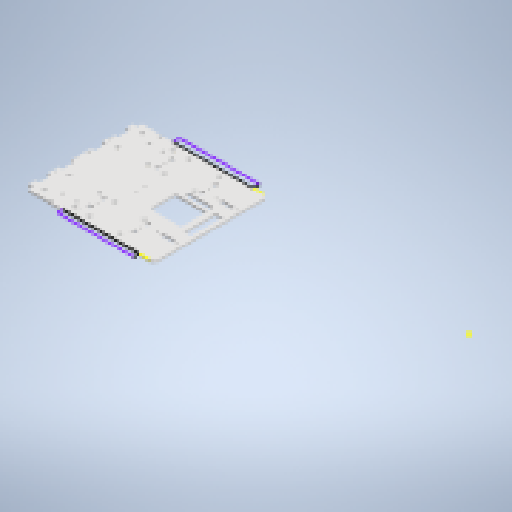
# Autodesk Inventor part: нижняя пластина
Saved by Autodesk Inventor 2024.2 (Build 282272000, 272)
## iProperties
Created: 2025-11-23
Part Number: нижняя пластина
Material: Типовые
Document SubType Name: Modeling
Designer: katya_notebook
Density: 1 g/cm^3
Appearance: По умолчанию
Author: katya_notebook
Autodesk Inventor part; units mm, degrees
(part 1 of 2)
ref_plane "YZ Plane" through (0, 0, 0) normal (1, 0, 0) x (0, 1, 0)
ref_plane "XZ Plane" through (0, 0, 0) normal (0, 1, 0) x (-1, 0, 0)
ref_plane "XY Plane" through (0, 0, 0) normal (0, 0, 1) x (1, 0, 0)
ref_plane "РабПлоскость1" through (-553.2789, -264.3002, 1.4222) normal (0, 1, 0) x (-1, 0, 0)
sketch "Эскиз1" plane through (-553.2789, -264.3002, 1.4222) normal (0, 1, 0) x (-1, 0, 0)
  line L0 (-30, 163.5) -> (30, 163.5) projected
  line L1 (-30, -31.5) -> (30, -31.5) projected
  line L2 (46.4763, 163.5) -> (-176.5237, 163.5)
  line L3 (-176.5237, 163.5) -> (-176.5237, -31.5)
  line L4 (-176.5237, -31.5) -> (46.4763, -31.5)
  line L5 (46.4763, -31.5) -> (46.4763, 163.5)
  point P0 (-553.2789, -1.4222)
  point P1 (-30, -30)
  point P2 (30, -30)
  point P3 (30, 162)
  point P4 (-30, 162)
  dimension "d23" = 8
  dimension "d24" = 8
  dimension "d1" = 223
  dimension "d6" = 0
  dimension "d7" = 0
  constraints: 8 end point, 2 coincident, 2 parallel, 1 horizontal, 1 perpendicular, 1 vertical
  measures "d1" distance of L2.start L2.end
  measures "d6" distance from line of L4 L1.end
  measures "d7" distance from line of L2 L0.end
extrude "Выдавливание1" add sketch "Эскиз1" along normal blind 4
sketch "Эскиз2" plane through (-553.2789, -264.3002, 1.4222) normal (0, -1, 0) x (1, 0, 0)
  circle A0 centre (26, 23.5) radius 2 projected
  circle A1 centre (-26, -19) radius 2 projected
  circle A2 centre (26, -19) radius 2
  circle A3 centre (-26, 23.5) radius 2 projected
  circle A4 centre (-26, -19) radius 2
  point P0 (553.2789, -1.4222)
  dimension "d23" = 8
  dimension "d24" = 8
  constraints: 2 centre point, 1 coincident, 1 concentric
extrude "Выдавливание2" cut sketch "Эскиз2" against normal blind 4
sketch "Эскиз7" plane through (-553.2789, -264.3002, 1.4222) normal (0, -1, 0) x (1, 0, 0)
  line L0 (30, 103.5) -> (30, 157) projected
  line L1 (-46.4763, 163.5) -> (176.5237, 163.5) projected
  line L2 (30.2701, 167.7701) -> (146.6973, 167.7701)
  line L3 (146.803, 163.5) -> (146.803, 157) projected
  line L4 (146.803, 167.7701) -> (146.6973, 167.7701)
  line L5 (146.803, 163.5) -> (30, 163.5)
  line L6 (30, 28.5) -> (30, -25) projected
  line L7 (30, -25) -> (30, -31.5) projected
  line L8 (146.803, -31.5) -> (146.803, -25) projected
  line L9 (146.803, -35.5) -> (30, -35.5)
  line L10 (30, -31.5) -> (146.803, -31.5)
  line L11 (30, 163.5) -> (26, 163.5)
  arc A0 (26, 163.5) -> (30.2701, 167.7701) centre (22.8966, 170.8735) ccw
  line L12 (146.803, 163.5) -> (150.803, 163.5)
  arc A1 (146.803, 167.7701) -> (150.803, 163.5) centre (154.2371, 170.7254) ccw
  line L13 (30, -31.5) -> (26, -31.5)
  line L14 (176.5237, -31.5) -> (-46.4763, -31.5) projected
  arc A2 (30, -35.5) -> (26, -31.5) centre (22.7085, -38.7915) ccw
  line L15 (146.803, -31.5) -> (150.803, -31.5)
  arc A3 (150.803, -31.5) -> (146.803, -35.5) centre (154.0945, -38.7915) ccw
  point P0 (553.2789, -1.4222)
  dimension "d23" = 8
  dimension "d24" = 8
  dimension "d26" = 8
  dimension "d28" = 8
  constraints: 18 end point, 8 point on circle, 5 point on line, 4 centre point, 2 collinear, 1 parallel
  measures "d23" radius of A0
  measures "d24" radius of A1
  measures "d26" radius of A2
  measures "d28" radius of A3
extrude "Выдавливание7" add sketch "Эскиз7" against normal blind 4
sketch "Эскиз10" plane through (-553.2789, -264.3002, 1.4222) normal (0, -1, 0) x (1, 0, 0)
  line L0 (36.9737, 147.85) -> (34.9737, 147.85)
  line L1 (36.9737, 147.85) -> (36.9737, 152.65)
  line L2 (35.9737, 147.85) -> (35.9737, 152.65)
  line L3 (36.9737, 159.35) -> (34.9737, 159.35)
  line L4 (36.9737, 150.25) -> (34.9737, 150.25)
  line L5 (36.9737, 159.35) -> (36.9737, 164.15)
  line L6 (36.9737, 161.75) -> (33.9943, 161.75)
  line L7 (33.9943, 161.75) -> (35.9737, 159.35)
  line L8 (35.9737, 164.15) -> (35.9737, 159.35)
  circle A0 centre (35.9737, 161.75) radius 1
  circle A1 centre (35.9737, 150.25) radius 1
  point P0 (553.2789, -1.4222)
  point P1 (34.9737, 147)
  point P2 (30, 163.5)
  point P3 (34.9737, 161.75)
  point P4 (35.9737, 162.75)
  point P5 (35.9737, 161.75)
  dimension "d23" = 8
  dimension "d24" = 8
  constraints: 18 end point, 4 midpoint, 4 perpendicular, 2 horizontal, 1 horizontal alignment, 6 other
extrude "Выдавливание10" cut sketch "Эскиз10" against normal blind 10 contours A1 L2 L4 | L4 L2 A1 | A1 L4 L2 | L4 A1 L2 | A0 L8 L6 | L6 L8 A0 | A0 L6 L8 | L6 A0 L8
sketch "Эскиз12" plane through (-553.2789, -264.3002, 1.4222) normal (0, -1, 0) x (1, 0, 0)
  circle A0 centre (55.5487, 57.8539) radius 2 projected
  circle A1 centre (55.5487, 73.8539) radius 2 projected
  point P0 (553.2789, -1.4222)
  dimension "d23" = 8
  dimension "d24" = 8
extrude "Выдавливание12" cut sketch "Эскиз12" against normal blind 10
sketch "Эскиз13" plane through (-553.2789, -264.3002, 1.4222) normal (0, -1, 0) x (1, 0, 0)
  point P0 (553.2789, -1.4222)
  dimension "d23" = 8
  dimension "d24" = 8
sketch "Эскиз15" plane through (-553.2789, -264.3002, 1.4222) normal (0, -1, 0) x (1, 0, 0)
  line L0 (169.5237, 93.5765) -> (157.5237, 93.5765)
  line L1 (157.5237, 93.5765) -> (157.5237, 38.5765)
  line L2 (157.5237, 38.5765) -> (169.5237, 38.5765)
  line L3 (169.5237, 38.5765) -> (169.5237, 93.5765)
  line L4 (169.5237, 93.5765) -> (157.5237, 38.5765) construction
  line L5 (157.5237, 93.5765) -> (169.5237, 38.5765) construction
  line L6 (176.5237, 163.5) -> (176.5237, -31.5) projected
  point P0 (553.2789, -1.4222)
  point P1 (163.5237, 66.0765)
  dimension "d23" = 8
  dimension "d24" = 8
  dimension "d57" = 13
  dimension "d58" = 12
  dimension "d59" = 55
  constraints: 12 end point, 2 midpoint, 2 parallel, 1 horizontal, 1 perpendicular
  measures "d57" distance from line of point (163.524, 66.076) L6
  measures "d58" distance of L0.start L0.end
  measures "d59" distance of L0.end L1.end
extrude "Выдавливание14" cut sketch "Эскиз15" against normal blind 10
sketch "Эскиз17" plane through (-553.2789, -260.3002, 1.4222) normal (0, 1, 0) x (1, 0, 0)
  line L0 (-46.4763, -143.5) -> (-46.4763, -123.5) projected
  line L1 (-46.4763, -143.5) -> (-40.4763, -143.5) projected
  line L2 (-40.4763, -123.5) -> (-40.4763, -143.5) projected
  line L3 (-46.4763, -123.5) -> (-40.4763, -123.5) projected
  line L4 (-46.4763, -103.5) -> (-46.4763, -83.5) projected
  line L5 (-46.4763, -103.5) -> (-40.4763, -103.5) projected
  line L6 (-40.4763, -83.5) -> (-40.4763, -103.5) projected
  line L7 (-46.4763, -83.5) -> (-40.4763, -83.5) projected
  line L8 (-46.4763, -48.5) -> (-46.4763, -28.5) projected
  line L9 (-46.4763, -48.5) -> (-40.4763, -48.5) projected
  line L10 (-40.4763, -28.5) -> (-40.4763, -48.5) projected
  line L11 (-46.4763, -28.5) -> (-40.4763, -28.5) projected
  line L12 (-46.4763, -8.5) -> (-46.4763, 11.5) projected
  line L13 (-46.4763, -8.5) -> (-40.4763, -8.5) projected
  line L14 (-40.4763, 11.5) -> (-40.4763, -8.5) projected
  line L15 (-46.4763, 11.5) -> (-40.4763, 11.5) projected
  circle A0 centre (-43.4763, -113.5) radius 1.75 projected
  circle A1 centre (-43.4763, -76.375) radius 1.75 projected
  circle A2 centre (-43.4763, -55.625) radius 1.75 projected
  circle A3 centre (-43.4763, -18.5) radius 1.75 projected
  point P0 (553.2789, 1.4222)
extrude "Выдавливание16" cut sketch "Эскиз17" against normal blind 10
fillet "Сопряжение1" radius 8 4 edges at (-376.7551, -262.3002, -30.0778) (-376.7551, -262.3002, 164.9222) (-599.7551, -262.3002, -30.0778) (-599.7551, -262.3002, 164.9222)
sketch "Эскиз18" plane through (-599.7551, -264.3002, 104.9222) normal (-1, 0, 0) x (0, 0, 1)
  line L0 (-95, 0) -> (-95, 4) projected
  line L1 (-95, 4) -> (-95, 5) projected
  line L2 (-95, 5) -> (-115, 5) projected
  line L3 (-115, 5) -> (-115, 4) projected
  line L4 (-135, 4) -> (-127, 4) projected
  line L5 (-135, 4) -> (-135, -55.705) projected
  line L6 (-115, -55.705) -> (-135, -55.705) projected
  line L7 (-115, -55.705) -> (-115, -60.705) projected
  line L8 (-115, -60.705) -> (-95, -60.705) projected
  line L9 (-95, -60.705) -> (-95, -55.705) projected
  line L10 (-86.75, -55.705) -> (-95, -55.705) projected
  line L11 (-86.75, -55.705) -> (-86.75, -54.205) projected
  line L12 (-86.75, -54.205) -> (-88.25, -54.205) projected
  line L13 (-88.25, -54.205) -> (-88.25, -51.205) projected
  line L14 (-88.25, -51.205) -> (-86.75, -51.205) projected
  line L15 (-86.75, -51.205) -> (-86.75, -43.705) projected
  line L16 (-86.75, -43.705) -> (-83.25, -43.705) projected
  line L17 (-83.25, -43.705) -> (-83.25, -51.205) projected
  line L18 (-83.25, -51.205) -> (-81.75, -51.205) projected
  line L19 (-81.75, -51.205) -> (-81.75, -54.205) projected
  line L20 (-81.75, -54.205) -> (-83.25, -54.205) projected
  line L21 (-83.25, -54.205) -> (-83.25, -55.705) projected
  line L22 (-75, -55.705) -> (-83.25, -55.705) projected
  line L23 (-75, -55.705) -> (-75, -60.705) projected
  line L24 (-75, -60.705) -> (-55, -60.705) projected
  line L25 (-55, -60.705) -> (-55, -55.705) projected
  line L26 (-49.625, -55.705) -> (-55, -55.705) projected
  line L27 (-49.625, -55.705) -> (-49.625, -54.205) projected
  line L28 (-49.625, -54.205) -> (-51.125, -54.205) projected
  line L29 (-51.125, -54.205) -> (-51.125, -51.205) projected
  line L30 (-51.125, -51.205) -> (-49.625, -51.205) projected
  line L31 (-49.625, -51.205) -> (-49.625, -49.705) projected
  line L32 (-49.625, -49.705) -> (-49.625, -49.705) projected
  line L33 (-49.625, -49.705) -> (-49.625, -43.705) projected
  line L34 (-49.625, -43.705) -> (-46.125, -43.705) projected
  line L35 (-46.125, -43.705) -> (-46.125, -51.205) projected
  line L36 (-46.125, -51.205) -> (-44.625, -51.205) projected
  line L37 (-44.625, -51.205) -> (-44.625, -54.205) projected
  line L38 (-44.625, -54.205) -> (-46.125, -54.205) projected
  line L39 (-46.125, -54.205) -> (-46.125, -55.705) projected
  line L40 (-28.875, -55.705) -> (-46.125, -55.705) projected
  line L41 (-28.875, -55.705) -> (-28.875, -54.205) projected
  line L42 (-28.875, -54.205) -> (-30.375, -54.205) projected
  line L43 (-30.375, -54.205) -> (-30.375, -51.205) projected
  line L44 (-30.375, -51.205) -> (-28.875, -51.205) projected
  line L45 (-28.875, -51.205) -> (-28.875, -43.705) projected
  line L46 (-28.875, -43.705) -> (-25.375, -43.705) projected
  line L47 (-25.375, -43.705) -> (-25.375, -51.205) projected
  line L48 (-25.375, -51.205) -> (-23.875, -51.205) projected
  line L49 (-23.875, -51.205) -> (-23.875, -54.205) projected
  line L50 (-23.875, -54.205) -> (-25.375, -54.205) projected
  line L51 (-25.375, -54.205) -> (-25.375, -55.705) projected
  line L52 (-20, -55.705) -> (-25.375, -55.705) projected
  line L53 (-20, -55.705) -> (-20, -60.705) projected
  line L54 (-20, -60.705) -> (0, -60.705) projected
  line L55 (0, -60.705) -> (0, -55.705) projected
  line L56 (8.25, -55.705) -> (0, -55.705) projected
  line L57 (8.25, -55.705) -> (8.25, -54.205) projected
  line L58 (8.25, -54.205) -> (6.75, -54.205) projected
  line L59 (6.75, -54.205) -> (6.75, -51.205) projected
  line L60 (6.75, -51.205) -> (8.25, -51.205) projected
  line L61 (8.25, -51.205) -> (8.25, -43.705) projected
  line L62 (8.25, -43.705) -> (11.75, -43.705) projected
  line L63 (11.75, -43.705) -> (11.75, -51.205) projected
  line L64 (11.75, -51.205) -> (13.25, -51.205) projected
  line L65 (13.25, -51.205) -> (13.25, -54.205) projected
  line L66 (13.25, -54.205) -> (11.75, -54.205) projected
  line L67 (11.75, -54.205) -> (11.75, -55.705) projected
  line L68 (20, -55.705) -> (11.75, -55.705) projected
  line L69 (20, -55.705) -> (20, -60.705) projected
  line L70 (20, -60.705) -> (40, -60.705) projected
  line L71 (40, -60.705) -> (40, -55.705) projected
  line L72 (60, -55.705) -> (40, -55.705) projected
  line L73 (60, 4) -> (60, -55.705) projected
  line L74 (52, 4) -> (60, 4) projected
  line L75 (40, 4) -> (40, 5) projected
  line L76 (40, 5) -> (20, 5) projected
  line L77 (20, 5) -> (20, 4) projected
  line L78 (20, 4) -> (20, 0) projected
  line L79 (20, 0) -> (13.25, 0) projected
  line L80 (13.25, 0) -> (13.25, -0.5) projected
  line L81 (13.25, -0.5) -> (11.75, -0.5) projected
  line L82 (11.75, -0.5) -> (11.75, -8) projected
  line L83 (11.75, -8) -> (8.25, -8) projected
  line L84 (8.25, -8) -> (8.25, -0.5) projected
  line L85 (8.25, -0.5) -> (6.75, -0.5) projected
  line L86 (6.75, -0.5) -> (6.75, 0) projected
  line L87 (6.75, 0) -> (0, 0) projected
  line L88 (0, 0) -> (0, 4) projected
  line L89 (0, 4) -> (0, 5) projected
  line L90 (0, 5) -> (-20, 5) projected
  line L91 (-20, 5) -> (-20, 4) projected
  line L92 (-20, 4) -> (-20, 0) projected
  line L93 (-20, 0) -> (-23.875, 0) projected
  line L94 (-23.875, 0) -> (-23.875, -0.5) projected
  line L95 (-23.875, -0.5) -> (-25.375, -0.5) projected
  line L96 (-25.375, -0.5) -> (-25.375, -8) projected
  line L97 (-25.375, -8) -> (-28.875, -8) projected
  line L98 (-28.875, -8) -> (-28.875, -0.5) projected
  line L99 (-28.875, -0.5) -> (-30.375, -0.5) projected
  line L100 (-30.375, -0.5) -> (-30.375, 0) projected
  line L101 (-30.375, 0) -> (-44.625, 0) projected
  line L102 (-44.625, 0) -> (-44.625, -0.5) projected
  line L103 (-44.625, -0.5) -> (-46.125, -0.5) projected
  line L104 (-46.125, -0.5) -> (-46.125, -8) projected
  line L105 (-46.125, -8) -> (-49.625, -8) projected
  line L106 (-49.625, -8) -> (-49.625, -2) projected
  line L107 (-49.625, -2) -> (-49.625, -2) projected
  line L108 (-49.625, -2) -> (-49.625, -0.5) projected
  line L109 (-49.625, -0.5) -> (-51.125, -0.5) projected
  line L110 (-51.125, -0.5) -> (-51.125, 0) projected
  line L111 (-51.125, 0) -> (-55, 0) projected
  line L112 (-55, 0) -> (-55, 4) projected
  line L113 (-55, 4) -> (-55, 5) projected
  line L114 (-55, 5) -> (-75, 5) projected
  line L115 (-75, 5) -> (-75, 4) projected
  line L116 (-75, 4) -> (-75, 0) projected
  line L117 (-75, 0) -> (-81.75, 0) projected
  line L118 (-81.75, 0) -> (-81.75, -0.5) projected
  line L119 (-81.75, -0.5) -> (-83.25, -0.5) projected
  line L120 (-83.25, -0.5) -> (-83.25, -8) projected
  line L121 (-83.25, -8) -> (-86.75, -8) projected
  line L122 (-86.75, -8) -> (-86.75, -0.5) projected
  line L123 (-86.75, -0.5) -> (-88.25, -0.5) projected
  line L124 (-88.25, -0.5) -> (-88.25, 0) projected
  line L125 (-88.25, 0) -> (-95, 0) projected
  line L126 (52, 0) -> (-127, 0) projected
  line L127 (52, 0) -> (52, 4)
  line L128 (52, 4) -> (60, 4)
  line L129 (60, 0) -> (60, 4)
  line L130 (60, 0) -> (52, 0)
  line L131 (-127, 0) -> (-127, 4)
  line L132 (-135, 0) -> (-135, 4)
  line L133 (-127, 4) -> (-135, 4)
  line L134 (-135, 0) -> (-127, 0)
  line L135 (-127, 0) -> (-127, 4) projected
  line L136 (52, 4) -> (52, 0) projected
  line L137 (52, 0) -> (40, 0) projected
  line L138 (40, 0) -> (40, 4) projected
  line L139 (-115, 4) -> (-115, 0) projected
  line L140 (-115, 0) -> (-127, 0) projected
  line L141 (-86.2339, -29.706) -> (-86.2339, -22.2488) projected
  spline S0 degree 2 poles (-86.2339, -22.2488) (-86.2339, -21.6567) (-85.6418, -21.6567) knots 0 0 0 1 1 1 projected
  spline S1 degree 2 poles (-85.6418, -21.6567) (-85.0497, -21.6567) (-85.0497, -22.2488) knots 0 0 0 1 1 1 projected
  line L142 (-85.0497, -22.2488) -> (-85.0497, -29.1139) projected
  line L143 (-85.0497, -29.1139) -> (-83.6248, -29.1139) projected
  line L144 (-83.6248, -29.1139) -> (-82.052, -22.0545) projected
  spline S2 degree 2 poles (-82.052, -22.0545) (-81.9595, -21.6567) (-81.4968, -21.6567) knots 0 0 0 1 1 1 projected
  spline S3 degree 2 poles (-81.4968, -21.6567) (-80.9047, -21.6567) (-80.9047, -22.2303) knots 0 0 0 1 1 1 projected
  spline S4 degree 2 poles (-80.9047, -22.2303) (-80.9047, -22.3043) (-80.914, -22.3599) knots 0 0 0 1 1 1 projected
  line L145 (-80.914, -22.3599) -> (-82.5886, -29.9003) projected
  spline S5 degree 2 poles (-82.5886, -29.9003) (-82.6811, -30.2889) (-83.153, -30.2889) knots 0 0 0 1 1 1 projected
  line L146 (-83.153, -30.2889) -> (-85.6418, -30.2889) projected
  spline S6 degree 2 poles (-85.6418, -30.2889) (-86.2339, -30.2889) (-86.2339, -29.706) knots 0 0 0 1 1 1 projected
  line L147 (-79.4429, -28.4663) -> (-79.4429, -23.4886) projected
  spline S7 degree 2 poles (-79.4429, -23.4886) (-79.4429, -22.7299) (-78.3696, -21.6567) (-77.611, -21.6567) knots 0 0 0 1 2 2 2 projected
  line L148 (-77.611, -21.6567) -> (-75.9548, -21.6567) projected
  spline S8 degree 2 poles (-75.9548, -21.6567) (-75.1869, -21.6567) (-74.1229, -22.7299) (-74.1229, -23.4886) knots 0 0 0 1 2 2 2 projected
  line L149 (-74.1229, -23.4886) -> (-74.1229, -28.4663) projected
  spline S9 degree 2 poles (-74.1229, -28.4663) (-74.1229, -29.2157) (-75.1962, -30.2889) (-75.9548, -30.2889) knots 0 0 0 1 2 2 2 projected
  line L150 (-75.9548, -30.2889) -> (-77.611, -30.2889) projected
  spline S10 degree 2 poles (-77.611, -30.2889) (-78.3604, -30.2889) (-79.4429, -29.2064) (-79.4429, -28.4663) knots 0 0 0 1 2 2 2 projected
  spline S11 degree 2 poles (-44.951, -30.2704) (-45.2008, -30.2704) (-45.5616, -29.9096) (-45.5616, -29.6783) knots 0 0 0 1 2 2 2 projected
  spline S12 degree 2 poles (-45.5616, -29.6783) (-45.5616, -29.4655) (-45.4043, -29.2897) knots 0 0 0 1 1 1 projected
  spline S13 degree 2 poles (-45.4043, -29.2897) (-44.109, -27.8649) (-42.8785, -26.5603) knots 0 0 0 1 1 1 projected
  line L151 (-42.8785, -26.5603) -> (-45.4506, -22.5542) projected
  spline S14 degree 2 poles (-45.4506, -22.5542) (-45.5431, -22.4061) (-45.5431, -22.2488) knots 0 0 0 1 1 1 projected
  spline S15 degree 2 poles (-45.5431, -22.2488) (-45.5431, -21.999) (-45.173, -21.6567) (-44.9417, -21.6567) knots 0 0 0 1 2 2 2 projected
  spline S16 degree 2 poles (-44.9417, -21.6567) (-44.6364, -21.6567) (-44.4328, -22.0638) knots 0 0 0 1 1 1 projected
  line L152 (-44.4328, -22.0638) -> (-42.1013, -25.7646) projected
  spline S17 degree 2 poles (-42.1013, -25.7646) (-42.0273, -25.5611) (-41.3982, -24.8672) knots 0 0 0 1 1 1 projected
  line L153 (-41.3982, -24.8672) -> (-41.3982, -22.2488) projected
  spline S18 degree 2 poles (-41.3982, -22.2488) (-41.3982, -21.6567) (-40.806, -21.6567) knots 0 0 0 1 1 1 projected
  spline S19 degree 2 poles (-40.806, -21.6567) (-40.2139, -21.6567) (-40.2139, -22.2488) knots 0 0 0 1 1 1 projected
  line L154 (-40.2139, -22.2488) -> (-40.2139, -29.706) projected
  spline S20 degree 2 poles (-40.2139, -29.706) (-40.2139, -30.2889) (-40.806, -30.2889) knots 0 0 0 1 1 1 projected
  spline S21 degree 2 poles (-40.806, -30.2889) (-41.3982, -30.2889) (-41.3982, -29.706) knots 0 0 0 1 1 1 projected
  line L155 (-41.3982, -29.706) -> (-41.3982, -26.3568) projected
  line L156 (-41.3982, -26.3568) -> (-44.4791, -29.9929) projected
  spline S22 degree 2 poles (-44.4791, -29.9929) (-44.7104, -30.2704) (-44.951, -30.2704) knots 0 0 0 1 1 1 projected
  line L157 (-33.6634, -29.7153) -> (-33.6634, -22.2488) projected
  spline S23 degree 2 poles (-33.6634, -22.2488) (-33.6634, -21.6567) (-33.0712, -21.6567) knots 0 0 0 1 1 1 projected
  line L158 (-33.0712, -21.6567) -> (-30.1753, -21.6567) projected
  spline S24 degree 2 poles (-30.1753, -21.6567) (-29.4074, -21.6567) (-28.3434, -22.7299) (-28.3434, -23.4979) knots 0 0 0 1 2 2 2 projected
  line L159 (-28.3434, -23.4979) -> (-28.3434, -29.7153) projected
  spline S25 degree 2 poles (-28.3434, -29.7153) (-28.3434, -30.2982) (-28.9355, -30.2982) knots 0 0 0 1 1 1 projected
  spline S26 degree 2 poles (-28.9355, -30.2982) (-29.5277, -30.2982) (-29.5277, -29.7153) knots 0 0 0 1 1 1 projected
  line L160 (-29.5277, -29.7153) -> (-29.5277, -23.4979) projected
  spline S27 degree 2 poles (-29.5277, -23.4979) (-29.5277, -23.2203) (-29.9163, -22.8317) (-30.1753, -22.8317) knots 0 0 0 1 2 2 2 projected
  line L161 (-30.1753, -22.8317) -> (-32.4791, -22.8317) projected
  line L162 (-32.4791, -22.8317) -> (-32.4791, -29.7153) projected
  spline S28 degree 2 poles (-32.4791, -29.7153) (-32.4791, -30.2982) (-33.0712, -30.2982) knots 0 0 0 1 1 1 projected
  spline S29 degree 2 poles (-33.0712, -30.2982) (-33.6634, -30.2982) (-33.6634, -29.7153) knots 0 0 0 1 1 1 projected
  line L163 (-26.8723, -29.706) -> (-26.8723, -22.2488) projected
  spline S30 degree 2 poles (-26.8723, -22.2488) (-26.8723, -21.6567) (-26.2802, -21.6567) knots 0 0 0 1 1 1 projected
  spline S31 degree 2 poles (-26.2802, -21.6567) (-25.6881, -21.6567) (-25.6881, -22.2488) knots 0 0 0 1 1 1 projected
  line L164 (-25.6881, -22.2488) -> (-25.6881, -29.706) projected
  spline S32 degree 2 poles (-25.6881, -29.706) (-25.6881, -30.2889) (-26.2802, -30.2889) knots 0 0 0 1 1 1 projected
  spline S33 degree 2 poles (-26.2802, -30.2889) (-26.8723, -30.2889) (-26.8723, -29.706) knots 0 0 0 1 1 1 projected
  line L165 (-19.2671, -28.4663) -> (-19.2671, -23.4886) projected
  spline S34 degree 2 poles (-19.2671, -23.4886) (-19.2671, -22.7392) (-18.1938, -21.6567) (-17.4167, -21.6567) knots 0 0 0 1 2 2 2 projected
  line L166 (-17.4167, -21.6567) -> (-15.779, -21.6567) projected
  spline S35 degree 2 poles (-15.779, -21.6567) (-15.0019, -21.6567) (-13.9286, -22.7299) (-13.9286, -23.4886) knots 0 0 0 1 2 2 2 projected
  line L167 (-13.9286, -23.4886) -> (-13.9286, -31.7878) projected
  spline S36 degree 2 poles (-13.9286, -31.7878) (-13.9286, -32.639) (-14.5022, -33.1386) knots 0 0 0 1 1 1 projected
  spline S37 degree 2 poles (-14.5022, -33.1386) (-15.0111, -33.6012) (-15.7605, -33.6012) knots 0 0 0 1 1 1 projected
  spline S38 degree 2 poles (-15.7605, -33.6012) (-16.5007, -33.6012) (-17.0188, -33.1386) knots 0 0 0 1 1 1 projected
  spline S39 degree 2 poles (-17.0188, -33.1386) (-17.5924, -32.6297) (-17.5924, -31.7785) knots 0 0 0 1 1 1 projected
  spline S40 degree 2 poles (-17.5924, -31.7785) (-17.5924, -31.1309) (-17.1668, -30.622) knots 0 0 0 1 1 1 projected
  spline S41 degree 2 poles (-17.1668, -30.622) (-16.8153, -30.3352) (-16.4637, -30.2889) knots 0 0 0 1 1 1 projected
  line L168 (-16.4637, -30.2889) -> (-17.4167, -30.2889) projected
  spline S42 degree 2 poles (-17.4167, -30.2889) (-18.1938, -30.2889) (-19.2671, -29.2157) (-19.2671, -28.4663) knots 0 0 0 1 2 2 2 projected
  line L169 (-12.476, -28.4663) -> (-12.476, -23.4886) projected
  spline S43 degree 2 poles (-12.476, -23.4886) (-12.476, -22.7299) (-11.4028, -21.6567) (-10.6441, -21.6567) knots 0 0 0 1 2 2 2 projected
  line L170 (-10.6441, -21.6567) -> (-8.988, -21.6567) projected
  spline S44 degree 2 poles (-8.988, -21.6567) (-8.22, -21.6567) (-7.1561, -22.7299) (-7.1561, -23.4886) knots 0 0 0 1 2 2 2 projected
  line L171 (-7.1561, -23.4886) -> (-7.1561, -28.4663) projected
  spline S45 degree 2 poles (-7.1561, -28.4663) (-7.1561, -29.2157) (-8.2293, -30.2889) (-8.988, -30.2889) knots 0 0 0 1 2 2 2 projected
  line L172 (-8.988, -30.2889) -> (-10.6441, -30.2889) projected
  spline S46 degree 2 poles (-10.6441, -30.2889) (-11.3935, -30.2889) (-12.476, -29.2064) (-12.476, -28.4663) knots 0 0 0 1 2 2 2 projected
  line L173 (1.0783, -28.4663) -> (1.0783, -23.4886) projected
  spline S47 degree 2 poles (1.0783, -23.4886) (1.0783, -22.7392) (2.1516, -21.6567) (2.9288, -21.6567) knots 0 0 0 1 2 2 2 projected
  line L174 (2.9288, -21.6567) -> (4.5664, -21.6567) projected
  spline S48 degree 2 poles (4.5664, -21.6567) (5.3436, -21.6567) (6.4168, -22.7299) (6.4168, -23.4886) knots 0 0 0 1 2 2 2 projected
  line L175 (6.4168, -23.4886) -> (6.4168, -31.7878) projected
  spline S49 degree 2 poles (6.4168, -31.7878) (6.4168, -32.639) (5.8432, -33.1386) knots 0 0 0 1 1 1 projected
  spline S50 degree 2 poles (5.8432, -33.1386) (5.3343, -33.6012) (4.5849, -33.6012) knots 0 0 0 1 1 1 projected
  spline S51 degree 2 poles (4.5849, -33.6012) (3.8447, -33.6012) (3.3266, -33.1386) knots 0 0 0 1 1 1 projected
  spline S52 degree 2 poles (3.3266, -33.1386) (2.753, -32.6297) (2.753, -31.7785) knots 0 0 0 1 1 1 projected
  spline S53 degree 2 poles (2.753, -31.7785) (2.753, -31.1309) (3.1786, -30.622) knots 0 0 0 1 1 1 projected
  spline S54 degree 2 poles (3.1786, -30.622) (3.5301, -30.3352) (3.8817, -30.2889) knots 0 0 0 1 1 1 projected
  line L176 (3.8817, -30.2889) -> (2.9288, -30.2889) projected
  spline S55 degree 2 poles (2.9288, -30.2889) (2.1516, -30.2889) (1.0783, -29.2157) (1.0783, -28.4663) knots 0 0 0 1 2 2 2 projected
  line L177 (14.6419, -29.706) -> (14.6419, -22.2488) projected
  spline S56 degree 2 poles (14.6419, -22.2488) (14.6419, -21.6567) (15.2341, -21.6567) knots 0 0 0 1 1 1 projected
  spline S57 degree 2 poles (15.2341, -21.6567) (15.8262, -21.6567) (15.8262, -22.2488) knots 0 0 0 1 1 1 projected
  line L178 (15.8262, -22.2488) -> (15.8262, -29.1139) projected
  line L179 (15.8262, -29.1139) -> (17.251, -29.1139) projected
  line L180 (17.251, -29.1139) -> (18.8239, -22.0545) projected
  spline S58 degree 2 poles (18.8239, -22.0545) (18.9164, -21.6567) (19.379, -21.6567) knots 0 0 0 1 1 1 projected
  spline S59 degree 2 poles (19.379, -21.6567) (19.9712, -21.6567) (19.9712, -22.2303) knots 0 0 0 1 1 1 projected
  spline S60 degree 2 poles (19.9712, -22.2303) (19.9712, -22.3043) (19.9619, -22.3599) knots 0 0 0 1 1 1 projected
  line L181 (19.9619, -22.3599) -> (18.2873, -29.9003) projected
  spline S61 degree 2 poles (18.2873, -29.9003) (18.1948, -30.2889) (17.7229, -30.2889) knots 0 0 0 1 1 1 projected
  line L182 (17.7229, -30.2889) -> (15.2341, -30.2889) projected
  spline S62 degree 2 poles (15.2341, -30.2889) (14.6419, -30.2889) (14.6419, -29.706) knots 0 0 0 1 1 1 projected
  line L183 (21.433, -30.9551) -> (21.433, -24.3213) projected
  spline S63 degree 2 poles (21.433, -24.3213) (21.433, -23.2111) (22.9966, -21.6567) (24.1069, -21.6567) knots 0 0 0 1 2 2 2 projected
  line L184 (24.1069, -21.6567) -> (24.9303, -21.6567) projected
  spline S64 degree 2 poles (24.9303, -21.6567) (26.0406, -21.6567) (27.5949, -23.2111) (27.5949, -24.3213) knots 0 0 0 1 2 2 2 projected
  line L185 (27.5949, -24.3213) -> (27.5949, -30.9551) projected
  spline S65 degree 2 poles (27.5949, -30.9551) (27.5949, -32.0561) (26.0406, -33.6104) (24.9303, -33.6104) knots 0 0 0 1 2 2 2 projected
  line L186 (24.9303, -33.6104) -> (24.1069, -33.6104) projected
  spline S66 degree 2 poles (24.1069, -33.6104) (22.9966, -33.6104) (21.433, -32.0561) (21.433, -30.9551) knots 0 0 0 1 2 2 2 projected
  line L187 (7.8694, -29.706) -> (7.8694, -22.2488) projected
  spline S67 degree 2 poles (7.8694, -22.2488) (7.8694, -21.6567) (8.4615, -21.6567) knots 0 0 0 1 1 1 projected
  line L188 (8.4615, -21.6567) -> (11.3574, -21.6567) projected
  spline S68 degree 2 poles (11.3574, -21.6567) (12.1254, -21.6567) (13.1894, -22.7299) (13.1894, -23.4886) knots 0 0 0 1 2 2 2 projected
  line L189 (13.1894, -23.4886) -> (13.1894, -29.706) projected
  spline S69 degree 2 poles (13.1894, -29.706) (13.1894, -30.2889) (12.5972, -30.2889) knots 0 0 0 1 1 1 projected
  spline S70 degree 2 poles (12.5972, -30.2889) (12.0051, -30.2889) (12.0051, -29.706) knots 0 0 0 1 1 1 projected
  line L190 (12.0051, -29.706) -> (12.0051, -23.4979) projected
  spline S71 degree 2 poles (12.0051, -23.4979) (12.0051, -23.2203) (11.6165, -22.8317) (11.3574, -22.8317) knots 0 0 0 1 2 2 2 projected
  line L191 (11.3574, -22.8317) -> (9.0537, -22.8317) projected
  line L192 (9.0537, -22.8317) -> (9.0537, -29.706) projected
  spline S72 degree 2 poles (9.0537, -29.706) (9.0537, -30.2889) (8.4615, -30.2889) knots 0 0 0 1 1 1 projected
  spline S73 degree 2 poles (8.4615, -30.2889) (7.8694, -30.2889) (7.8694, -29.706) knots 0 0 0 1 1 1 projected
  spline S74 degree 2 poles (-5.1113, -30.2704) (-5.3611, -30.2704) (-5.722, -29.9096) (-5.722, -29.6783) knots 0 0 0 1 2 2 2 projected
  spline S75 degree 2 poles (-5.722, -29.6783) (-5.722, -29.4655) (-5.5647, -29.2897) knots 0 0 0 1 1 1 projected
  spline S76 degree 2 poles (-5.5647, -29.2897) (-4.2694, -27.8649) (-3.0389, -26.5603) knots 0 0 0 1 1 1 projected
  line L193 (-3.0389, -26.5603) -> (-5.6109, -22.5542) projected
  spline S77 degree 2 poles (-5.6109, -22.5542) (-5.7035, -22.4061) (-5.7035, -22.2488) knots 0 0 0 1 1 1 projected
  spline S78 degree 2 poles (-5.7035, -22.2488) (-5.7035, -21.999) (-5.3334, -21.6567) (-5.1021, -21.6567) knots 0 0 0 1 2 2 2 projected
  spline S79 degree 2 poles (-5.1021, -21.6567) (-4.7968, -21.6567) (-4.5932, -22.0638) knots 0 0 0 1 1 1 projected
  line L194 (-4.5932, -22.0638) -> (-2.2617, -25.7646) projected
  spline S80 degree 2 poles (-2.2617, -25.7646) (-2.1877, -25.5611) (-1.5585, -24.8672) knots 0 0 0 1 1 1 projected
  line L195 (-1.5585, -24.8672) -> (-1.5585, -22.2488) projected
  spline S81 degree 2 poles (-1.5585, -22.2488) (-1.5585, -21.6567) (-0.9664, -21.6567) knots 0 0 0 1 1 1 projected
  spline S82 degree 2 poles (-0.9664, -21.6567) (-0.3742, -21.6567) (-0.3742, -22.2488) knots 0 0 0 1 1 1 projected
  line L196 (-0.3742, -22.2488) -> (-0.3742, -29.706) projected
  spline S83 degree 2 poles (-0.3742, -29.706) (-0.3742, -30.2889) (-0.9664, -30.2889) knots 0 0 0 1 1 1 projected
  spline S84 degree 2 poles (-0.9664, -30.2889) (-1.5585, -30.2889) (-1.5585, -29.706) knots 0 0 0 1 1 1 projected
  line L197 (-1.5585, -29.706) -> (-1.5585, -26.3568) projected
  line L198 (-1.5585, -26.3568) -> (-4.6395, -29.9929) projected
  spline S85 degree 2 poles (-4.6395, -29.9929) (-4.8708, -30.2704) (-5.1113, -30.2704) knots 0 0 0 1 1 1 projected
  line L199 (-25.2162, -24.7377) -> (-25.2162, -23.4886) projected
  spline S86 degree 2 poles (-25.2162, -23.4886) (-25.2162, -22.7299) (-24.1429, -21.6567) (-23.375, -21.6567) knots 0 0 0 1 2 2 2 projected
  line L200 (-23.375, -21.6567) -> (-21.3025, -21.6567) projected
  spline S87 degree 2 poles (-21.3025, -21.6567) (-20.7104, -21.6567) (-20.7104, -22.2488) knots 0 0 0 1 1 1 projected
  line L201 (-20.7104, -22.2488) -> (-20.7104, -29.706) projected
  spline S88 degree 2 poles (-20.7104, -29.706) (-20.7104, -30.2889) (-21.3025, -30.2889) knots 0 0 0 1 1 1 projected
  spline S89 degree 2 poles (-21.3025, -30.2889) (-21.8947, -30.2889) (-21.8947, -29.706) knots 0 0 0 1 1 1 projected
  line L202 (-21.8947, -29.706) -> (-21.8947, -26.5603) projected
  line L203 (-21.8947, -26.5603) -> (-23.3843, -26.5603) projected
  spline S90 degree 2 poles (-23.3843, -26.5603) (-24.1429, -26.5603) (-25.2162, -25.4778) (-25.2162, -24.7377) knots 0 0 0 1 2 2 2 projected
  spline S91 degree 2 poles (-32.4143, -33.0276) (-32.4143, -32.4354) (-31.8222, -32.4354) knots 0 0 0 1 1 1 projected
  line L204 (-31.8222, -32.4354) -> (-30.1846, -32.4354) projected
  spline S92 degree 2 poles (-30.1846, -32.4354) (-29.5924, -32.4354) (-29.5924, -33.0276) knots 0 0 0 1 1 1 projected
  spline S93 degree 2 poles (-29.5924, -33.0276) (-29.5924, -33.6104) (-30.1846, -33.6104) knots 0 0 0 1 1 1 projected
  line L205 (-30.1846, -33.6104) -> (-31.8222, -33.6104) projected
  spline S94 degree 2 poles (-31.8222, -33.6104) (-32.4143, -33.6104) (-32.4143, -33.0276) knots 0 0 0 1 1 1 projected
  spline S95 degree 2 poles (-52.6765, -22.7762) (-53.0836, -22.6189) (-53.0836, -22.2396) knots 0 0 0 1 1 1 projected
  spline S96 degree 2 poles (-53.0836, -22.2396) (-53.0836, -21.6289) (-52.5007, -21.6289) knots 0 0 0 1 1 1 projected
  spline S97 degree 2 poles (-52.5007, -21.6289) (-52.0658, -21.6289) (-51.631, -22.2118) knots 0 0 0 1 1 1 projected
  spline S98 degree 2 poles (-51.631, -22.2118) (-51.2239, -21.6567) (-50.3912, -21.6567) knots 0 0 0 1 1 1 projected
  line L206 (-50.3912, -21.6567) -> (-48.7351, -21.6567) projected
  spline S99 degree 2 poles (-48.7351, -21.6567) (-47.9672, -21.6567) (-46.9032, -22.7299) (-46.9032, -23.4886) knots 0 0 0 1 2 2 2 projected
  line L207 (-46.9032, -23.4886) -> (-46.9032, -28.4663) projected
  spline S100 degree 2 poles (-46.9032, -28.4663) (-46.9032, -29.2157) (-47.9764, -30.2889) (-48.7351, -30.2889) knots 0 0 0 1 2 2 2 projected
  line L208 (-48.7351, -30.2889) -> (-51.631, -30.2889) projected
  spline S101 degree 2 poles (-51.631, -30.2889) (-52.2231, -30.2889) (-52.2231, -29.706) knots 0 0 0 1 1 1 projected
  line L209 (-52.2231, -29.706) -> (-52.2231, -23.4701) projected
  spline S102 degree 2 poles (-52.2231, -23.4701) (-52.2231, -22.9612) (-52.6765, -22.7762) knots 0 0 0 1 1 1 projected
  line L210 (-59.0975, -28.4663) -> (-59.0975, -23.4886) projected
  spline S103 degree 2 poles (-59.0975, -23.4886) (-59.0975, -22.7392) (-58.0242, -21.6567) (-57.2563, -21.6567) knots 0 0 0 1 2 2 2 projected
  line L211 (-57.2563, -21.6567) -> (-55.6187, -21.6567) projected
  spline S104 degree 2 poles (-55.6187, -21.6567) (-54.8415, -21.6567) (-53.7775, -22.7299) (-53.7775, -23.4886) knots 0 0 0 1 2 2 2 projected
  line L212 (-53.7775, -23.4886) -> (-53.7775, -28.4663) projected
  spline S105 degree 2 poles (-53.7775, -28.4663) (-53.7775, -29.2157) (-54.8415, -30.2889) (-55.6187, -30.2889) knots 0 0 0 1 2 2 2 projected
  line L213 (-55.6187, -30.2889) -> (-56.5716, -30.2889) projected
  line L214 (-56.5716, -30.2889) -> (-54.0828, -32.5557) projected
  spline S106 degree 2 poles (-54.0828, -32.5557) (-53.722, -32.824) (-53.722, -33.0923) knots 0 0 0 1 1 1 projected
  spline S107 degree 2 poles (-53.722, -33.0923) (-53.722, -33.6104) (-54.3696, -33.6104) knots 0 0 0 1 1 1 projected
  line L215 (-54.3696, -33.6104) -> (-58.5053, -33.6104) projected
  spline S108 degree 2 poles (-58.5053, -33.6104) (-59.0975, -33.6104) (-59.0975, -33.0276) knots 0 0 0 1 1 1 projected
  spline S109 degree 2 poles (-59.0975, -33.0276) (-59.0975, -32.4354) (-58.5053, -32.4354) knots 0 0 0 1 1 1 projected
  line L216 (-58.5053, -32.4354) -> (-55.5632, -32.4354) projected
  line L217 (-55.5632, -32.4354) -> (-58.6349, -29.632) projected
  spline S110 degree 2 poles (-58.6349, -29.632) (-59.0975, -29.2157) (-59.0975, -28.4663) knots 0 0 0 1 1 1 projected
  line L218 (-64.0566, -21.6474) -> (-61.7436, -21.6474) projected
  line L219 (-61.7436, -21.6474) -> (-61.7436, -18.9273) projected
  spline S111 degree 2 poles (-61.7436, -18.9273) (-61.7436, -18.3352) (-61.1514, -18.3352) knots 0 0 0 1 1 1 projected
  spline S112 degree 2 poles (-61.1514, -18.3352) (-60.5593, -18.3352) (-60.5593, -18.9273) knots 0 0 0 1 1 1 projected
  line L220 (-60.5593, -18.9273) -> (-60.5593, -29.706) projected
  spline S113 degree 2 poles (-60.5593, -29.706) (-60.5593, -30.2889) (-61.1514, -30.2889) knots 0 0 0 1 1 1 projected
  line L221 (-61.1514, -30.2889) -> (-64.0566, -30.2889) projected
  spline S114 degree 2 poles (-64.0566, -30.2889) (-64.806, -30.2889) (-65.8793, -29.2157) (-65.8793, -28.4755) knots 0 0 0 1 2 2 2 projected
  line L222 (-65.8793, -28.4755) -> (-65.8793, -23.4886) projected
  spline S115 degree 2 poles (-65.8793, -23.4886) (-65.8793, -22.7392) (-64.806, -21.6474) (-64.0566, -21.6474) knots 0 0 0 1 2 2 2 projected
  line L223 (-72.6611, -29.706) -> (-72.6611, -22.2488) projected
  spline S116 degree 2 poles (-72.6611, -22.2488) (-72.6611, -21.6567) (-72.0689, -21.6567) knots 0 0 0 1 1 1 projected
  line L224 (-72.0689, -21.6567) -> (-69.173, -21.6567) projected
  spline S117 degree 2 poles (-69.173, -21.6567) (-68.4051, -21.6567) (-67.3411, -22.7299) (-67.3411, -23.4886) knots 0 0 0 1 2 2 2 projected
  line L225 (-67.3411, -23.4886) -> (-67.3411, -29.706) projected
  spline S118 degree 2 poles (-67.3411, -29.706) (-67.3411, -30.2889) (-67.9332, -30.2889) knots 0 0 0 1 1 1 projected
  spline S119 degree 2 poles (-67.9332, -30.2889) (-68.5254, -30.2889) (-68.5254, -29.706) knots 0 0 0 1 1 1 projected
  line L226 (-68.5254, -29.706) -> (-68.5254, -23.4979) projected
  spline S120 degree 2 poles (-68.5254, -23.4979) (-68.5254, -23.2203) (-68.914, -22.8317) (-69.173, -22.8317) knots 0 0 0 1 2 2 2 projected
  line L227 (-69.173, -22.8317) -> (-71.4768, -22.8317) projected
  line L228 (-71.4768, -22.8317) -> (-71.4768, -29.706) projected
  spline S121 degree 2 poles (-71.4768, -29.706) (-71.4768, -30.2889) (-72.0689, -30.2889) knots 0 0 0 1 1 1 projected
  spline S122 degree 2 poles (-72.0689, -30.2889) (-72.6611, -30.2889) (-72.6611, -29.706) knots 0 0 0 1 1 1 projected
  line L229 (-92.4051, -25.3853) -> (-88.8708, -25.3853) projected
  line L230 (-88.8708, -25.3853) -> (-88.8708, -23.4886) projected
  spline S123 degree 2 poles (-88.8708, -23.4886) (-88.8708, -23.2111) (-89.2501, -22.8317) (-89.5092, -22.8317) knots 0 0 0 1 2 2 2 projected
  line L231 (-89.5092, -22.8317) -> (-92.4051, -22.8317) projected
  spline S124 degree 2 poles (-92.4051, -22.8317) (-92.9972, -22.8317) (-92.9972, -22.2488) knots 0 0 0 1 1 1 projected
  spline S125 degree 2 poles (-92.9972, -22.2488) (-92.9972, -21.6567) (-92.4051, -21.6567) knots 0 0 0 1 1 1 projected
  line L232 (-92.4051, -21.6567) -> (-89.5092, -21.6567) projected
  spline S126 degree 2 poles (-89.5092, -21.6567) (-88.7413, -21.6567) (-87.6865, -22.7299) (-87.6865, -23.4886) knots 0 0 0 1 2 2 2 projected
  line L233 (-87.6865, -23.4886) -> (-87.6865, -28.4663) projected
  spline S127 degree 2 poles (-87.6865, -28.4663) (-87.6865, -29.2064) (-88.7505, -30.2889) (-89.5092, -30.2889) knots 0 0 0 1 2 2 2 projected
  line L234 (-89.5092, -30.2889) -> (-91.1746, -30.2889) projected
  spline S128 degree 2 poles (-91.1746, -30.2889) (-91.9332, -30.2889) (-93.0065, -29.2157) (-93.0065, -28.457) knots 0 0 0 1 2 2 2 projected
  line L235 (-93.0065, -28.457) -> (-93.0065, -25.9774) projected
  spline S129 degree 2 poles (-93.0065, -25.9774) (-93.0065, -25.3853) (-92.4051, -25.3853) knots 0 0 0 1 1 1 projected
  line L236 (-97.7898, -22.2488) -> (-97.7898, -29.1139) projected
  line L237 (-97.7898, -29.1139) -> (-95.6526, -29.1139) projected
  line L238 (-95.6526, -29.1139) -> (-95.6526, -22.2488) projected
  spline S130 degree 2 poles (-95.6526, -22.2488) (-95.6526, -21.6567) (-95.0605, -21.6567) knots 0 0 0 1 1 1 projected
  spline S131 degree 2 poles (-95.0605, -21.6567) (-94.4683, -21.6567) (-94.4683, -22.2488) knots 0 0 0 1 1 1 projected
  line L239 (-94.4683, -22.2488) -> (-94.4683, -29.706) projected
  spline S132 degree 2 poles (-94.4683, -29.706) (-94.4683, -30.2889) (-95.0605, -30.2889) knots 0 0 0 1 1 1 projected
  line L240 (-95.0605, -30.2889) -> (-100.4544, -30.2889) projected
  spline S133 degree 2 poles (-100.4544, -30.2889) (-101.2131, -30.2889) (-102.2956, -29.2064) (-102.2956, -28.4663) knots 0 0 0 1 2 2 2 projected
  line L241 (-102.2956, -28.4663) -> (-102.2956, -22.2488) projected
  spline S134 degree 2 poles (-102.2956, -22.2488) (-102.2956, -21.6567) (-101.7035, -21.6567) knots 0 0 0 1 1 1 projected
  spline S135 degree 2 poles (-101.7035, -21.6567) (-101.1113, -21.6567) (-101.1113, -22.2488) knots 0 0 0 1 1 1 projected
  line L242 (-101.1113, -22.2488) -> (-101.1113, -28.457) projected
  spline S136 degree 2 poles (-101.1113, -28.457) (-101.1113, -28.7253) (-100.7228, -29.1139) (-100.4544, -29.1139) knots 0 0 0 1 2 2 2 projected
  line L243 (-100.4544, -29.1139) -> (-98.9741, -29.1139) projected
  line L244 (-98.9741, -29.1139) -> (-98.9741, -22.2488) projected
  spline S137 degree 2 poles (-98.9741, -22.2488) (-98.9741, -21.6567) (-98.382, -21.6567) knots 0 0 0 1 1 1 projected
  spline S138 degree 2 poles (-98.382, -21.6567) (-97.7898, -21.6567) (-97.7898, -22.2488) knots 0 0 0 1 1 1 projected
  point P0 (-104.9222, 264.3002)
  constraints: 16 end point, 6 perpendicular, 4 point on line, 2 parallel, 1 other
extrude "Выдавливание17" cut sketch "Эскиз18" against normal blind 8 contours L134 L5 L4 L131 | L127 L74 L73 L130